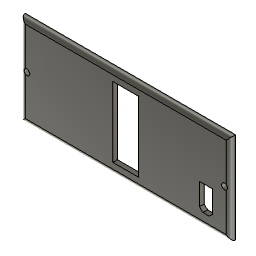
untere heckplatte (Autodesk Fusion 360 design; units mm, degrees)
Autodesk Fusion 360 part; units mm, degrees
sketch "Skizze1" plane through (0, 0, 0) normal (0, 1, 0) x (1, 0, 0)
  line L0 (0, 0) -> (90, 0)
  line L1 (90, 0) -> (90, -39)
  line L2 (90, -39) -> (0, -39)
  line L3 (0, -39) -> (0, 0)
  line L4 (0, -39) -> (2.75, -39)
  line L5 (90, -39) -> (87.25, -39)
  line L6 (2.75, -39) -> (2.75, -19.5)
  line L7 (87.25, -39) -> (87.25, -19.5)
  circle A0 centre (2.75, -19.5) radius 1.25
  circle A1 centre (87.25, -19.5) radius 1.25
  dimension "d1" = 39
  dimension "d2" = 90
  dimension "d3" = 2.75
  dimension "d4" = 2.75
  dimension "d5" = 19.5
  dimension "d6" = 19.5
  dimension "d7" = 2.5
  dimension "d8" = 2.5
  constraint horizontal L0
  constraint vertical L1
  constraint horizontal L2
  constraint vertical L3
  constraint coincident L0.start L3.end
  constraint perpendicular L3 L4
  constraint perpendicular L1 L5
  constraint perpendicular L4 L6
  constraint perpendicular L2 L7
  constraint coincident L6.end A0.centre
  constraint coincident L7.end A1.centre
  measures "d1" distance of L0.start L2.end
  measures "d2" distance of L1.end L2.end
  measures "d3" distance of L2.end L4.end
  measures "d4" distance of L1.end L5.end
  measures "d5" distance of L4.end L6.end
  measures "d6" distance of L5.end L7.end
  measures "d7" diameter of A0
  measures "d8" diameter of A1
extrude "Extrusion1" add sketch "Skizze1" along normal blind 3
fillet "Abrundung1" radius 2 4 edges at (90, 0, 19.5) (45, 0, 39) (45, 0, 0) (0, 0, 19.5)
extrude "Extrusion2" cut 1 faces at (58.6969, 3, 6.3442) along direction (0, -1, 0) blind 1
sketch "Skizze2" plane through (0, 0, 0) normal (0, -1, 0) x (1, 0, 0)
  line L0 (88, 20.5) -> (88, 37)
  line L1 (88, 37) -> (2, 37)
  line L2 (2, 37) -> (2, 20.5)
  arc A0 (2, 18.5) -> (2, 20.5) centre (2.75, 19.5) ccw
  line L3 (2, 18.5) -> (2, 2)
  line L4 (2, 2) -> (88, 2)
  line L5 (88, 2) -> (88, 18.5)
  arc A1 (88, 20.5) -> (88, 18.5) centre (87.25, 19.5) ccw
  line L6 (2.75, 19.5) -> (45, 19.5)
  line L7 (50.5, 34.5) -> (39.5, 34.5)
  line L8 (39.5, 34.5) -> (39.5, 4.5)
  line L9 (39.5, 4.5) -> (50.5, 4.5)
  line L10 (50.5, 4.5) -> (50.5, 34.5)
  line L11 (50.5, 34.5) -> (39.5, 4.5) construction
  line L12 (39.5, 34.5) -> (50.5, 4.5) construction
  point P0 (45, 19.5)
  dimension "d15" = 42.25
  dimension "d16" = 11
  dimension "d17" = 30
  constraint coincident A0.centre L6.start
  constraint perpendicular L0 L6
  constraint horizontal L7
  constraint perpendicular L7 L8
  constraint parallel L7 L9
  constraint parallel L8 L10
  constraint coincident L11 P0
  constraint coincident L12 P0
  constraint coincident P0 L6.end
  measures "d15" distance of A0.centre P0
  measures "d16" distance of L8.end L9.end
  measures "d17" distance of L7.end L8.end
extrude "Extrusion3" cut sketch "Skizze2" against normal blind 8 contours L7 L8 L9 L10
sketch "Skizze3" plane through (0, 0, 0) normal (0, -1, 0) x (1, 0, 0)
  line L0 (39.5, 34.5) -> (50.5, 34.5)
  line L1 (50.5, 34.5) -> (50.5, 4.5)
  line L2 (50.5, 4.5) -> (39.5, 4.5)
  line L3 (39.5, 4.5) -> (39.5, 34.5)
  line L4 (88, 20.5) -> (88, 37)
  line L5 (88, 37) -> (2, 37)
  line L6 (2, 37) -> (2, 20.5)
  arc A0 (2, 18.5) -> (2, 20.5) centre (2.75, 19.5) ccw
  line L7 (2, 18.5) -> (2, 2)
  line L8 (2, 2) -> (88, 2)
  line L9 (88, 2) -> (88, 18.5)
  arc A1 (88, 20.5) -> (88, 18.5) centre (87.25, 19.5) ccw
  line L10 (90, 0) -> (79.3979, 10.6111)
  line L11 (76.5979, 16.0111) -> (82.1979, 16.0111)
  line L12 (82.1979, 16.0111) -> (82.1979, 5.2111)
  line L13 (82.1979, 5.2111) -> (76.5979, 5.2111)
  line L14 (76.5979, 5.2111) -> (76.5979, 16.0111)
  line L15 (76.5979, 16.0111) -> (82.1979, 5.2111) construction
  line L16 (82.1979, 16.0111) -> (76.5979, 5.2111) construction
  line L17 (76.5979, 5.2111) -> (77.305, 5.9182)
  line L18 (76.5979, 5.2111) -> (77.5979, 5.2111) construction
  line L19 (77.305, 5.9182) -> (76.5979, 6.6253)
  line L20 (77.305, 5.9182) -> (78.0121, 5.2111)
  line L21 (82.1979, 5.2111) -> (81.4908, 5.9182)
  line L22 (81.4908, 5.9182) -> (82.1979, 6.6253)
  line L23 (81.4908, 5.9182) -> (80.7837, 5.2111)
  point P0 (79.3979, 10.6111)
  dimension "d22" = 15
  dimension "d23" = 5.6
  dimension "d24" = 10.8
  dimension "d25" = 45
  dimension "d26" = 1
  dimension "d27" = 1
  constraint horizontal L11
  constraint perpendicular L11 L12
  constraint parallel L11 L13
  constraint parallel L12 L14
  constraint coincident L15 P0
  constraint coincident L16 P0
  constraint coincident P0 L10.end
  constraint horizontal L18
  constraint coincident L14 L19.end
  constraint perpendicular L17 L19
  constraint coincident L13 L20.end
  constraint perpendicular L17 L20
  constraint parallel L20 L21
  constraint coincident L12 L22.end
  constraint perpendicular L21 L22
  constraint coincident L13 L23.end
  constraint perpendicular L21 L23
  measures "d22" distance of L10.start P0
  measures "d23" distance of L12.end L13.end
  measures "d24" distance of L11.end L12.end
  measures "d25" angle of L17 L18
  measures "d26" distance of L13.end L17.end
  measures "d27" distance of L12.end L21.end
extrude "Extrusion4" cut sketch "Skizze3" against normal blind 122 contours L11 L12 L13 L14 L19 L20 L22 L23
